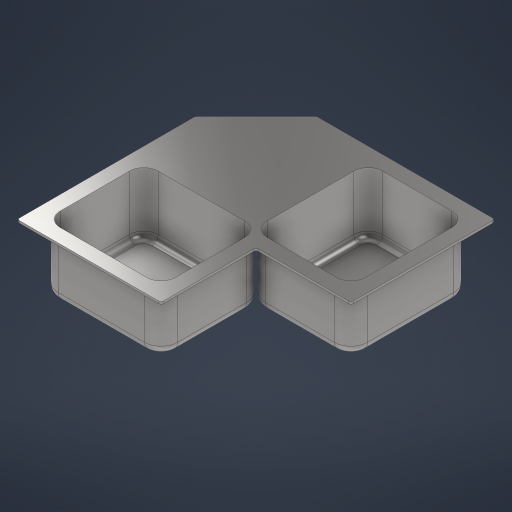
# Autodesk Inventor part: Lavandino ad angolo Apell ROAN2IBC
Saved by Autodesk Inventor 2024.2 (Build 282272000, 272)
## iProperties
Created: 2025-08-23
Part Number: Lavandino ad angolo Apell ROAN2IBC
Material: Iron, Malleable
Document SubType Name: Modeling
Designer: Luca
Density: 7.15 g/cm^3
Appearance: Semi-Polished
Author: Luca
Autodesk Inventor part; units mm, degrees
ref_plane "YZ Plane" through (0, 0, 0) normal (1, 0, 0) x (0, 1, 0)
ref_plane "XZ Plane" through (0, 0, 0) normal (0, 1, 0) x (-1, 0, 0)
sketch "Sketch1" plane through (0, 0, 0) normal (0, 1, 0) x (-1, 0, 0)
  line L0 (0, 0) -> (0, 330)
  line L1 (0, 330) -> (500, 330)
  line L2 (500, 330) -> (500, -287.868)
  line L3 (500, -287.868) -> (287.868, -500)
  line L4 (287.868, -500) -> (-330, -500)
  line L5 (-330, -500) -> (-330, 0)
  line L6 (-330, 0) -> (0, 0)
  dimension "d0" = 500
  dimension "d1" = 830
  dimension "d2" = 300
  constraints: 14 end point, 7 perpendicular, 1 parallel, 1 vertical
  measures "d0" distance of L4.end L5.end
  measures "d1" distance between parallel lines of L5 L2
  measures "d2" distance of L2.end L3.end
extrude "Extrusion1" add sketch "Sketch1" against normal blind 8
sketch "Sketch2" plane through (0, -8, 0) normal (0, -1, 0) x (1, 0, 0)
  line L0 (-100, 280) -> (-400, 280) construction
  line L1 (-450, 230) -> (-450, -10) construction
  line L2 (-400, -60) -> (-100, -60) construction
  line L3 (-50, -10) -> (-50, 230) construction
  line L4 (230, -50) -> (-10, -50) construction
  line L5 (-60, -100) -> (-60, -400) construction
  line L6 (-10, -450) -> (230, -450) construction
  line L7 (280, -400) -> (280, -100) construction
  line L8 (330, 0) -> (0, 0) projected
  line L9 (330, -500) -> (330, 0) projected
  line L10 (0, 0) -> (0, 330) projected
  line L11 (0, 330) -> (-500, 330) projected
  arc A0 (-50, 230) -> (-100, 280) centre (-100, 230) ccw construction
  arc A1 (-100, -60) -> (-50, -10) centre (-100, -10) ccw construction
  arc A2 (-10, -50) -> (-60, -100) centre (-10, -100) ccw construction
  arc A3 (-60, -400) -> (-10, -450) centre (-10, -400) ccw construction
  arc A4 (230, -450) -> (280, -400) centre (230, -400) ccw construction
  arc A5 (280, -100) -> (230, -50) centre (230, -100) ccw construction
  arc A6 (-450, -10) -> (-400, -60) centre (-400, -10) ccw construction
  arc A7 (-400, 280) -> (-450, 230) centre (-400, 230) ccw construction
  line L12 (-42, -10) -> (-42, 230)
  arc A8 (-42, 230) -> (-100, 288) centre (-100, 230) ccw
  line L13 (-100, 288) -> (-400, 288)
  arc A9 (-400, 288) -> (-458, 230) centre (-400, 230) ccw
  line L14 (-458, 230) -> (-458, -10)
  arc A10 (-458, -10) -> (-400, -68) centre (-400, -10) ccw
  line L15 (-400, -68) -> (-100, -68)
  arc A11 (-100, -68) -> (-42, -10) centre (-100, -10) ccw
  line L16 (-68, -100) -> (-68, -400)
  arc A12 (-68, -400) -> (-10, -458) centre (-10, -400) ccw
  line L17 (-10, -458) -> (230, -458)
  arc A13 (230, -458) -> (288, -400) centre (230, -400) ccw
  line L18 (288, -400) -> (288, -100)
  arc A14 (288, -100) -> (230, -42) centre (230, -100) ccw
  line L19 (230, -42) -> (-10, -42)
  arc A15 (-10, -42) -> (-68, -100) centre (-10, -100) ccw
  point P0 (-450, -60)
  point P1 (-450, 280)
  point P2 (-50, -60)
  point P3 (280, -250)
  dimension "d5" = 400
  dimension "d6" = 340
  dimension "d7" = 250
  dimension "d8" = 50
  dimension "d9" = 50
  dimension "d10" = 50
  dimension "d11" = 50
  dimension "d12" = 8
  dimension "d13" = 8
  constraints: 32 end point, 32 point on circle, 16 centre point, 16 tangent, 8 parallel, 7 equal radius, 6 perpendicular, 6 point on line, 2 horizontal, 1 midpoint, 14 other
  measures "d5" distance of point (-50, -60) point (-450, -60)
  measures "d6" distance of point (-450, -60) point (-450, 280)
  measures "d7" distance from line of point (280, -250) L8
  measures "d8" distance between parallel lines of L9 L7
  measures "d9" distance between parallel lines of L3 L10
  measures "d10" distance between parallel lines of L11 L0
  measures "d11" radius of A0
  measures "d12" distance between parallel lines of L15 L2
  measures "d13" distance between parallel lines of L5 L16
extrude "Extrusion2" add sketch "Sketch2" along normal blind 213
fillet "Fillet1" radius 30 16 edges at (-68, -221, -250) (-51.0122, -221, -441.0122) (110, -221, -458) (271.0122, -221, -441.0122) (288, -221, -250) (271.0122, -221, -58.9878) (110, -221, -42) (-51.0122, -221, -58.9878) (-58.9878, -221, 271.0122) (-250, -221, 288) (-441.0122, -221, 271.0122) (-458, -221, 110) (-441.0122, -221, -51.0122) (-250, -221, -68) (-58.9878, -221, -51.0122) (-42, -221, 110)
shell "Shell1" thickness 8 removed faces 1 at (14.044, 0, -333.3333)
ref_plane "Work Plane1" through (0, 0, 0) normal (0.7071068, 0, -0.7071068) x (0, -1, 0)
fillet "Fillet2" radius 8 7 edges at (-500, -4, 330) (0, -4, 330) (330, -4, 0) (0, -4, 0) (-500, -4, -287.868) (-287.868, -4, -500) (330, -4, -500)
body "Solid1"
